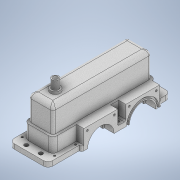
# Autodesk Inventor part: Gehäuse oben
Saved by Autodesk Inventor 2022 (Build 260153000, 153)
## iProperties
Created: 2023-01-26
Part Number: Gehäuse oben
Material: Aluminium 6061
Document SubType Name: Modeling
Designer: Matias Nicky
Density: 2.7 g/cm^3
Appearance: Aluminiumguss
Author: Matias Nicky
Autodesk Inventor part; units mm, degrees
ref_plane "YZ Plane" through (0, 0, 0) normal (1, 0, 0) x (0, 1, 0)
ref_plane "XZ Plane" through (0, 0, 0) normal (0, 1, 0) x (-1, 0, 0)
ref_plane "XY Plane" through (0, 0, 0) normal (0, 0, 1) x (1, 0, 0)
sketch "Skizze1" plane through (0, 0, 0) normal (0, 1, 0) x (-1, 0, 0)
  line L0 (-20, -102) -> (20, -102)
  line L1 (25, -97) -> (25, 97)
  line L2 (20, 102) -> (-20, 102)
  line L3 (-25, 97) -> (-25, -97)
  line L4 (-25, -102) -> (25, 102) construction
  line L5 (25, -102) -> (-25, 102) construction
  arc A0 (-20, 102) -> (-25, 97) centre (-20, 97) ccw
  arc A1 (25, 97) -> (20, 102) centre (20, 97) ccw
  arc A2 (20, -102) -> (25, -97) centre (20, -97) ccw
  arc A3 (-25, -97) -> (-20, -102) centre (-20, -97) ccw
  point P0 (0, 0)
  dimension "d0" = 50
  dimension "d1" = 204
  dimension "d8" = 5
  constraints: 12 end point, 8 point on circle, 8 point on line, 8 tangent, 4 centre point, 3 equal radius, 2 midpoint, 2 parallel, 1 horizontal, 1 perpendicular
  measures "d0" distance of L5.end L4.end
  measures "d1" distance of L4.end L5.start
  measures "d8" radius of A0
extrude "Extrusion1" add sketch "Skizze1" along normal blind 93
sketch "Skizze2" plane through (0, 0, 0) normal (0, -1, 0) x (1, 0, 0)
  line L0 (-15, 97) -> (15, 97)
  line L1 (20, 92) -> (20, -92)
  line L2 (15, -97) -> (-15, -97)
  line L3 (-20, -92) -> (-20, 92)
  line L4 (-20, 97) -> (20, -97) construction
  line L5 (20, 97) -> (-20, -97) construction
  arc A0 (20, 92) -> (15, 97) centre (15, 92) ccw
  arc A1 (-15, 97) -> (-20, 92) centre (-15, 92) ccw
  arc A2 (-20, -92) -> (-15, -97) centre (-15, -92) ccw
  arc A3 (15, -97) -> (20, -92) centre (15, -92) ccw
  point P0 (0, 0)
  dimension "d4" = 40
  dimension "d5" = 194
  dimension "d9" = 5
  constraints: 12 end point, 8 point on circle, 8 point on line, 8 tangent, 4 centre point, 3 equal radius, 2 midpoint, 2 parallel, 1 horizontal, 1 perpendicular
  measures "d4" distance of L4.end L5.end
  measures "d5" distance of L5.start L4.end
  measures "d9" radius of A0
extrude "Extrusion2" cut sketch "Skizze2" against normal blind 85
sketch "Skizze3" plane through (0, 0, 0) normal (0, -1, 0) x (1, 0, 0)
  line L0 (-20, 102) -> (20, 102)
  line L1 (25, 97) -> (25, -97)
  line L2 (20, -102) -> (-20, -102)
  line L3 (-25, -97) -> (-25, 97)
  line L4 (-25, 102) -> (25, -102) construction
  line L5 (25, 102) -> (-25, -102) construction
  arc A0 (25, 97) -> (20, 102) centre (20, 97) ccw
  arc A1 (20, -102) -> (25, -97) centre (20, -97) ccw
  arc A2 (-25, -97) -> (-20, -102) centre (-20, -97) ccw
  arc A3 (-20, 102) -> (-25, 97) centre (-20, 97) ccw
  line L6 (-40, 127) -> (40, 127)
  line L7 (40, -127) -> (-40, -127)
  line L8 (-40, 127) -> (40, -127) construction
  line L9 (40, 127) -> (-40, -127) construction
  line L10 (40, 127) -> (40, 62.597)
  line L11 (45, -104.403) -> (40, -104.403)
  line L12 (40, -104.403) -> (40, -127)
  line L13 (-40, -127) -> (-40, -104.403)
  line L14 (-40, -104.403) -> (-45, -104.403)
  line L15 (-45, -104.403) -> (-45, -24.403)
  line L16 (-45, -17.403) -> (-45, 62.597)
  line L17 (-45, 62.597) -> (-40, 62.597)
  line L18 (-40, 62.597) -> (-40, 127)
  line L19 (45, -24.403) -> (45, -64.403)
  line L20 (45, -64.403) -> (45, -104.403)
  line L21 (15, -97) -> (-15, -97) projected
  line L22 (45, 62.597) -> (40, 62.597)
  line L23 (45, -17.403) -> (45, 22.597)
  line L24 (45, 22.597) -> (45, 62.597)
  line L25 (-63, 0) -> (63, 0) projected
  line L26 (-45, -24.403) -> (-45, -17.403)
  line L27 (45, -24.403) -> (45, -17.403)
  point P0 (0, 0)
  dimension "d20" = 0
  dimension "d10" = 5
  dimension "d11" = 80
  dimension "d12" = 254
  dimension "d17" = 32.597
  dimension "d24" = 80
  dimension "d25" = 87
  dimension "d53" = 80
  dimension "d151" = 7.403
  dimension "d254" = 5
  dimension "d255" = 5
  constraints: 52 end point, 19 point on line, 10 vertical, 8 point on circle, 8 tangent, 6 equal length, 6 horizontal, 5 perpendicular, 4 centre point, 4 midpoint, 3 collinear, 3 equal radius, 17 other
  measures "d10" radius of A0
  measures "d11" distance of L8.end L9.end
  measures "d12" distance of L9.start L8.end
  measures "d17" distance from line of L19.end L21
  measures "d24" distance of L23.start L22.start
  measures "d25" distance of L23.end L19.end
  measures "d53" distance of L16.start L16.end
  measures "d151" distance between parallel lines of L21 L14
  measures "d254" distance between parallel lines of L13 L15
  measures "d255" distance between parallel lines of L18 L16
fillet "Rundung1" radius 5 8 edges at (18.5355, 85, 95.5355) (20, 85, 0) (18.5355, 85, -95.5355) (0, 85, -97) (-18.5355, 85, -95.5355) (-20, 85, 0) (-18.5355, 85, 95.5355) (0, 85, 97)
extrude "Extrusion3" add sketch "Skizze3" against normal blind 40 contours A3 L3 L25 L16 L17 L18 L6 L10 L22 L24 L23 L1 A0 L0 | L3 A2 L2 A1 L1 L25 L23 L27 L19 L20 L11 L12 L7 L13 L14 L15 L26 L16
sketch "Skizze13" plane through (45, 0, 62.597) normal (1, 0, 0) x (0, 0, -1)
  circle A0 centre (127, 0) radius 24.5
  line L0 (167, 0) -> (0, 0) projected
  circle A1 centre (40, 0) radius 24.5
  point P0 (159.597, 0)
  point P1 (15.5, 0)
  point P2 (64.5, 0)
  point P3 (102.5, 0)
  point P4 (151.5, 0)
  dimension "d74" = 49
  dimension "d75" = 32.597
  dimension "d78" = 87
  constraints: 2 centre point, 1 equal radius, 1 point on line
  measures "d74" diameter of A0
  measures "d75" distance of A0.centre point (159.597, 0)
  measures "d78" distance of A1.centre A0.centre
extrude "Extrusion12" cut sketch "Skizze13" against normal through all contours L0 A0 | L0 A1 picked at (133.1128, 9.3243) picked at (41.2217, 10.0615)
sketch "Skizze15" plane through (45, 0, -104.403) normal (1, 0, 0) x (0, 0, -1)
  arc A0 (-15.5, 0) -> (-64.5, 0) centre (-40, 0) ccw projected
  circle A1 centre (-40, 0) radius 27.5
  point P0 (-104.403, 0)
  dimension "d85" = 55
  constraints: 1 centre point, 1 coincident
  measures "d85" diameter of A1
extrude "Extrusion14" cut sketch "Skizze15" against normal blind 22
sketch "Skizze16" plane through (-45, 0, 62.597) normal (-1, 0, 0) x (0, 0, 1)
  arc A0 (-15.5, 0) -> (-64.5, 0) centre (-40, 0) ccw projected
  circle A1 centre (-40, 0) radius 27.5
  point P0 (-62.597, 0)
  dimension "d88" = 55
  constraints: 1 centre point, 1 coincident
  measures "d88" diameter of A1
extrude "Extrusion15" cut sketch "Skizze16" against normal blind 22
sketch "Skizze17" plane through (-45, 0, 62.597) normal (-1, 0, 0) x (0, 0, 1)
  arc A0 (-102.5, 0) -> (-151.5, 0) centre (-127, 0) ccw projected
  circle A1 centre (-127, 0) radius 27.5
  point P0 (-62.597, 0)
  dimension "d91" = 55
  constraints: 1 centre point, 1 coincident
  measures "d91" diameter of A1
extrude "Extrusion16" cut sketch "Skizze17" against normal blind 20
sketch "Skizze18" plane through (45, 0, -104.403) normal (1, 0, 0) x (0, 0, -1)
  arc A0 (-102.5, 0) -> (-151.5, 0) centre (-127, 0) ccw projected
  circle A1 centre (-127, 0) radius 27.5
  point P0 (-104.403, 0)
  dimension "d94" = 55
  constraints: 1 centre point, 1 coincident
  measures "d94" diameter of A1
extrude "Extrusion17" cut sketch "Skizze18" against normal blind 20
sketch "Skizze20" plane through (-45, 0, 62.597) normal (-1, 0, 0) x (0, 0, 1)
  arc A0 (-99.5, 0) -> (-154.5, 0) centre (-127, 0) ccw projected
  arc A1 (-12.5, 0) -> (-67.5, 0) centre (-40, 0) ccw projected
  circle A2 centre (-40, 0) radius 30
  circle A3 centre (-40, 0) radius 33.55
  dimension "d106" = 60
  dimension "d107" = 67.1
  constraints: 2 centre point, 2 coincident
  measures "d106" diameter of A2
  measures "d107" diameter of A3
extrude "Extrusion20" cut sketch "Skizze20" against normal blind 3.55
sketch "Skizze21" plane through (45, 0, -104.403) normal (1, 0, 0) x (0, 0, -1)
  circle A0 centre (-40, 0) radius 30
  arc A1 (-15.5, 0) -> (-64.5, 0) centre (-40, 0) ccw projected
  circle A2 centre (-40, 0) radius 33.55
  point P0 (-104.403, 0)
  point P1 (-40, 0)
  dimension "d110" = 60
  dimension "d111" = 67.1
  constraints: 2 centre point, 2 coincident
  measures "d110" diameter of A0
  measures "d111" diameter of A2
extrude "Extrusion21" cut sketch "Skizze21" against normal blind 3.55
fillet "Rundung4" radius 10 4 edges at (-40, 20, -127) (40, 20, -127) (-40, 20, 127) (40, 20, 127)
fillet "Rundung5" radius 10 8 edges at (-23.5355, 93, 100.5355) (0, 93, 102) (23.5355, 93, 100.5355) (25, 93, 0) (23.5355, 93, -100.5355) (0, 93, -102) (-23.5355, 93, -100.5355) (-25, 93, 0)
sketch "Skizze22" plane through (0, 40, 0) normal (0, 1, 0) x (1, 0, 0)
  arc A0 (40, 117) -> (30, 127) centre (30, 117) ccw projected
  arc A1 (-30, 127) -> (-40, 117) centre (-30, 117) ccw projected
  line L0 (30, 127) -> (-30, 127)
  line L1 (-30, 127) -> (-40, 127)
  line L2 (-40, 117) -> (-40, 104.403) projected
  line L3 (-40, 127) -> (-40, 104.403)
  line L4 (-45, 104.403) -> (-40, 104.403) projected
  line L5 (-40, 104.403) -> (-45, 104.403)
  line L6 (-45, 104.403) -> (-45, 99.403)
  line L7 (-45, 91.903) -> (-45, 104.403) projected
  line L8 (-45, 99.403) -> (-30, 99.403)
  line L9 (-30, 99.403) -> (-30, 107)
  line L10 (-30, 107) -> (30, 107)
  line L11 (30, 107) -> (30, 99.403)
  line L12 (30, 99.403) -> (45, 99.403)
  line L13 (45, 99.403) -> (45, 104.403)
  line L14 (45, 104.403) -> (40, 104.403) projected
  line L15 (45, 104.403) -> (40, 104.403)
  line L16 (40, 117) -> (40, 104.403) projected
  line L17 (40, 104.403) -> (40, 117)
  line L18 (40, 117) -> (40, 127)
  line L19 (40, 127) -> (30, 127)
  line L20 (45, -62.597) -> (45, 104.403) projected
  line L21 (45, 29.403) -> (30, 29.403)
  line L22 (30, 29.403) -> (30, 12.403)
  line L23 (30, 12.403) -> (45, 12.403)
  line L24 (45, 12.403) -> (45, 29.403)
  line L25 (45, -62.597) -> (45, -57.597)
  line L26 (45, -57.597) -> (30, -57.597)
  line L27 (30, -57.597) -> (30, -107)
  line L28 (30, -107) -> (-30, -107)
  line L29 (-30, -107) -> (-30, -57.597)
  line L30 (-30, -57.597) -> (-45, -57.597)
  line L31 (-45, -57.597) -> (-45, -62.597)
  line L32 (-45, -62.597) -> (-40, -62.597)
  arc A2 (-40, -117) -> (-30, -127) centre (-30, -117) ccw projected
  line L33 (-40, -62.597) -> (-40, -117)
  line L34 (-40, -117) -> (-40, -127)
  line L35 (-40, -127) -> (-30, -127)
  line L36 (-30, -127) -> (30, -127)
  line L37 (40, -127) -> (40, -117)
  line L38 (40, -117) -> (40, -62.597) projected
  line L39 (40, -117) -> (40, -62.597)
  line L40 (-30, 29.403) -> (-45, 29.403)
  line L41 (40, -62.597) -> (45, -62.597) projected
  line L42 (45, -62.597) -> (40, -62.597)
  line L43 (-30, 29.403) -> (-30, 12.403)
  line L44 (-30, 12.403) -> (-45, 12.403)
  line L45 (-45, 12.403) -> (-45, 29.403)
  line L46 (30, -127) -> (40, -127)
  point P0 (0, 0)
  point P1 (-45, 4.903)
  dimension "d117" = 5
  dimension "d118" = 20
  dimension "d119" = 15
  dimension "d120" = 15
  dimension "d121" = 5
  dimension "d122" = 70
  dimension "d123" = 5
  dimension "d124" = 20
  dimension "d126" = 15
  dimension "d128" = 15
  dimension "d131" = 70
  dimension "d132" = 70
  dimension "d136" = 70
  constraints: 80 end point, 19 perpendicular, 11 point on line, 6 tangent, 4 horizontal, 3 vertical, 2 collinear, 2 parallel
  measures "d117" distance of L4.start L6.end
  measures "d118" distance between parallel lines of L0 L10
  measures "d119" distance of L11.end L12.end
  measures "d120" distance of L6.end L8.end
  measures "d121" distance of L12.end L13.end
  measures "d122" distance between parallel lines of L12 L21
  measures "d123" distance of L20.start L25.end
  measures "d124" distance between parallel lines of L36 L28
  measures "d126" distance between parallel lines of L27 L20
  measures "d128" distance of L29.end L30.end
  measures "d131" distance between parallel lines of L26 L23
  measures "d132" distance between parallel lines of L8 L40
  measures "d136" distance between parallel lines of L44 L30
extrude "Extrusion22" cut sketch "Skizze22" against normal blind 30 contours L16 L14 L13 L12 L11 L10 L9 L8 L6 L4 L2 A1 L0 A0 | L41 L38 L37 L46 L36 A2 L33 L32 L31 L30 L29 L28 L27 L26 L20 | L23 L22 L21 L20 | L43 L44 L45 L40
sketch "Skizze23" plane through (0, 0, 0) normal (0, -1, 0) x (1, 0, 0)
  line L0 (-20, -39.903) -> (-20, -1.903) projected
  line L1 (-30, -29.403) -> (-30, -12.403) projected
  line L2 (-30, -12.403) -> (-45, -12.403) projected
  line L3 (-30, -127) -> (30, -127) projected
  line L4 (30, 127) -> (-30, 127) projected
  line L5 (45, -30.853) -> (45, -4.903) projected
  line L6 (45, -12.403) -> (30, -12.403) projected
  line L7 (0, -177.8) -> (0, 177.8) projected
  point P0 (0, 0)
  point P1 (-15, -117)
  point P2 (15, -117)
  point P3 (-20, -4.903)
  point P4 (-15, 117)
  point P5 (15, 117)
  dimension "d137" = 10
  dimension "d139" = 10
  dimension "d140" = 10
  dimension "d146" = 30
  dimension "d147" = 15
  dimension "d148" = 30
  dimension "d149" = 10
  dimension "d150" = 15
  measures "d137" distance from line of L3 point (-15, -117)
  measures "d139" distance from line of L3 point (15, -117)
  measures "d140" distance from line of L4 point (15, 117)
  measures "d146" distance of point (15, -117) point (-15, -117)
  measures "d147" distance from line of L7 point (15, -117)
  measures "d148" distance of point (15, 117) point (-15, 117)
  measures "d149" distance from line of L4 point (-15, 117)
  measures "d150" distance from line of point (15, 117) L7
hole "Bohrung1" at (-15, 0, -117) at (15, 0, -117) at (-15, 0, 117) at (15, 0, 117) direction (0, 1, 0) diameter 8.376 depth 27.3 thread size "M10x1.5" class "6H" standard "ANSI Metric M Profile"
fillet "Rundung6" radius 10 4 edges at (30, 25, 107) (-30, 25, 107) (-30, 25, -107) (30, 25, -107)
sketch "Skizze24" plane through (0, 0, 0) normal (0, -1, 0) x (1, 0, 0)
  line L0 (-40, 117) -> (-40, 62.597) projected
  line L1 (-45, 50.097) -> (-23, 50.097) projected
  line L2 (40, 62.597) -> (40, 117) projected
  line L3 (25, 50.097) -> (45, 50.097) projected
  line L4 (45, -91.903) -> (23, -91.903) projected
  line L5 (40, -117) -> (40, -104.403) projected
  line L6 (-40, -104.403) -> (-40, -117) projected
  line L7 (-25, -91.903) -> (-45, -91.903) projected
  line L8 (45, -30.853) -> (45, -4.903) projected
  line L9 (41.45, -30.853) -> (45, -30.853) projected
  line L10 (45, -12.403) -> (30, -12.403) projected
  line L11 (-45, -10.953) -> (-45, -36.903) projected
  line L12 (15, -97) -> (-15, -97) projected
  line L13 (-15, 97) -> (15, 97) projected
  point P0 (0, 0)
  point P1 (-35, 65.097)
  point P2 (-33.5, 107)
  point P3 (-20, 50.097)
  point P4 (33.5, 107)
  point P5 (35, 65.097)
  point P6 (33.5, -107)
  point P7 (20, -91.903)
  point P8 (-33.5, -107)
  point P9 (37.5, -20.903)
  point P10 (-45, -12.403)
  dimension "d161" = 6.5
  dimension "d162" = 5
  dimension "d163" = 15
  dimension "d172" = 6.5
  dimension "d173" = 5
  dimension "d174" = 15
  dimension "d176" = 6.5
  dimension "d177" = 6.5
  dimension "d192" = 10
  dimension "d193" = 10
  dimension "d194" = 10
  measures "d161" distance from line of L0 point (-33.5, 107)
  measures "d162" distance from line of L0 point (-35, 65.097)
  measures "d163" distance from line of L1 point (-35, 65.097)
  measures "d172" distance from line of L2 point (33.5, 107)
  measures "d173" distance from line of L2 point (35, 65.097)
  measures "d174" distance from line of L3 point (35, 65.097)
  measures "d176" distance from line of point (33.5, -107) L5
  measures "d177" distance from line of L6 point (-33.5, -107)
  measures "d192" distance from line of point (-33.5, -107) L12
  measures "d193" distance from line of point (33.5, -107) L12
  measures "d194" distance from line of point (-33.5, 107) L13
hole "Bohrung3" at (-35, 0, 65.097) at (-33.5, 0, 107) at (33.5, 0, 107) at (35, 0, 65.097) at (33.5, 0, -107) at (-33.5, 0, -107) direction (0, 1, 0) diameter 4.134 depth 14.2 thread size "M5x0.8" class "6H" standard "ANSI Metric M Profile"
fillet "Rundung7" radius 3 4 edges at (37.5, 10, -12.403) (37.5, 10, -29.403) (-37.5, 10, -12.403) (-37.5, 10, -29.403)
sketch "Skizze25" plane through (0, 0, 0) normal (0, -1, 0) x (1, 0, 0)
  line L0 (-45, -10.953) -> (-45, -36.903) projected
  line L1 (45, -30.853) -> (45, -4.903) projected
  line L2 (45, -15.403) -> (30, -15.403) projected
  line L3 (-30, -15.403) -> (-45, -15.403) projected
  point P0 (0, 0)
  point P1 (-37.5, -20.903)
  point P2 (37.5, -20.903)
  point P3 (-45, -12.403)
  point P4 (45, -12.403)
  dimension "d195" = 7.5
  dimension "d196" = 7.5
  dimension "d206" = 8.5
  dimension "d207" = 8.5
  measures "d195" distance from line of L0 point (-37.5, -20.903)
  measures "d196" distance from line of L1 point (37.5, -20.903)
  measures "d206" vertical distance of point (-37.5, -20.903) point (-45, -12.403)
  measures "d207" vertical distance of point (45, -12.403) point (37.5, -20.903)
hole "Bohrung4" at (37.5, 0, -20.903) at (-37.5, 0, -20.903) direction (0, 1, 0) diameter 4.917 depth 17.1 thread size "M6x1" class "6H" standard "ANSI Metric M Profile"
sketch "Skizze26" plane through (45, 0, 62.597) normal (1, 0, 0) x (0, 0, -1)
  line L0 (92, 40) -> (162, 40) projected
  line L1 (162, 10) -> (162, 40) projected
  line L2 (92, 40) -> (92, 13) projected
  line L3 (5, 40) -> (75, 40) projected
  line L4 (75, 13) -> (75, 40) projected
  line L5 (5, 40) -> (5, 10) projected
  point P0 (62.597, 0)
  point P1 (155, 33)
  point P2 (99, 33)
  point P3 (68, 33)
  point P4 (12, 33)
  dimension "d208" = 7
  dimension "d209" = 7
  dimension "d210" = 7
  dimension "d211" = 7
  dimension "d212" = 7
  dimension "d213" = 7
  dimension "d214" = 7
  dimension "d215" = 7
  measures "d208" distance from line of L0 point (155, 33)
  measures "d209" distance from line of L1 point (155, 33)
  measures "d210" distance from line of L0 point (99, 33)
  measures "d211" distance from line of L2 point (99, 33)
  measures "d212" distance from line of L3 point (68, 33)
  measures "d213" distance from line of L4 point (68, 33)
  measures "d214" distance from line of L3 point (12, 33)
  measures "d215" distance from line of L5 point (12, 33)
hole "Bohrung5" at (45, 33, -92.403) at (45, 33, -36.403) at (45, 33, -5.403) at (45, 33, 50.597) direction (-1, 0, 0) diameter 4.134 depth 14.2 thread size "M5x0.8" class "6H" standard "ANSI Metric M Profile"
sketch "Skizze27" plane through (-45, 0, -104.403) normal (-1, 0, 0) x (0, 0, 1)
  circle A0 centre (155, 33) radius 2.067 projected
  circle A1 centre (99, 33) radius 2.067 projected
  circle A2 centre (68, 33) radius 2.067 projected
  circle A3 centre (12, 33) radius 2.067 projected
  point P0 (104.403, 0)
  constraints: 4 coincident
hole "Bohrung6" at (-45, 33, 50.597) at (-45, 33, -5.403) at (-45, 33, -36.403) at (-45, 33, -92.403) direction (1, 0, 0) diameter 4.134 depth 14.2 thread size "M5x0.8" class "6H" standard "ANSI Metric M Profile"
fillet "Rundung8" radius 5 4 edges at (-45, 5, 62.597) (-45, 5, -104.403) (45, 5, -104.403) (45, 5, 62.597)
sketch "Skizze28" plane through (0, 93, 0) normal (0, 1, 0) x (1, 0, 0)
  circle A0 centre (0, -72) radius 10
  line L0 (15, -92) -> (-15, -92) projected
  point P0 (0, 0)
  dimension "d231" = 20
  dimension "d232" = 20
  constraints: 1 centre point
  measures "d231" diameter of A0
  measures "d232" distance from line of L0 A0.centre
extrude "Extrusion23" add sketch "Skizze28" along normal blind 5
sketch "Skizze29" plane through (0, 98, 72) normal (0, 1, 0) x (1, 0, 0)
  circle A0 centre (0, 0) radius 7
  point P0 (0, 72)
  dimension "d242" = 14
  constraints: 1 centre point
  measures "d242" diameter of A0
extrude "Extrusion24" add sketch "Skizze29" along normal blind 18
thread "Gewinde1" size "M14x2" class "6g" standard "ANSI Metric M Profile" length 29.966
sketch "Skizze30" plane through (0, 116, 72) normal (0, 1, 0) x (1, 0, 0)
  point P0 (0, 72)
  point P1 (0, 0)
hole "Bohrung8" at (0, 116, 72) direction (0, -1, 0) diameter 10 end through all
